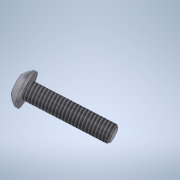
# Autodesk Inventor part: SCREW, BUTTON HD, P, 12.9, M4X0.7X18MM
Saved by Autodesk Inventor 2024.2 (Build 282272000, 272)
## iProperties
Manager: 100-31865
Category: _
Created: 2013-04-09
Material: Steel
Description: SCREW, BUTTON HD, P, 12.9, M4X0.7X18MM
Document SubType Name: Modeling
Designer: robr , Rob
Checked By: 2ATE9
Engr Approved By: R
User Status: Released
Density: 7.85 g/cm^3
Mfg Approved By: Rob.Roddy
Appearance: Plate
Part Number: SCREW, BUTTON HD, P, 12.9, M4X0.7X18MM
Mass: 2.32497 g
Surface Area: 3.53377 cm^2
Volume: 0.296174 cm^3
Control State: 0
Master: False
Checked Out: False
Shininess: 65.0
Length Units: 11269
Angle Units: 11279
Time Units: 11290
Mass Units: 11286
Length Display Precision: 4
Angle Display Precision: 2
Compacted: True
CN_SERVICEABLE: _
CN_MASS: 0.002378
CL_runCount: 1
FinishProperty: ToBeSet
FIRST_DESCRIPTION: SCREW, BUTTON HD, P, 12.9, M4X0.7X18MM
SECOND_DESCRIPTION: _
THIRD_DESCRIPTION: _
CN_DETAILER: -
CN_MFG_PART_NUM: FMPBHMA040070018
CN_MFG_NAME: -
STANDARDCLASSFLAG: R
CUSTOMERNUMBER: _
CN_DESIGNER: Rob.Roddy
PTC_WM_ITERATION: 3
PTC_WM_ORGANIZATION_ID: CLWC
PTC_WM_LIFECYCLE: CLWC_CAD_LC
Density: 7.86
Volumn: 1.0470389527034538
Area: 8.192112949038872
PropertySet Name: Model Information
Revision Number: 1
Subject: FMPBHMA040070018
Author: -
Keywords: -
Autodesk Inventor part; units mm, degrees
ref_plane "YZ Plane" through (0, 0, 0) normal (1, 0, 0) x (0, 1, 0)
ref_plane "XZ Plane" through (0, 0, 0) normal (0, 1, 0) x (-1, 0, 0)
ref_plane "XY Plane" through (0, 0, 0) normal (0, 0, 1) x (1, 0, 0)
sketch "Sketch1" plane through (0, 0, 0) normal (0, 0, 1) x (1, 0, 0)
  line L0 (0, -22.0606) -> (0, 6.3638) projected
  line L1 (0, 2.2) -> (2.25, 2.2)
  line L2 (3.8, 0) -> (3.8, 0.56)
  arc A0 (3.8, 0.56) -> (2.25, 2.2) centre (0, -1.479) ccw
  line L3 (3.8, 0) -> (2, 0)
  line L4 (2, 0) -> (2, -10)
  line L5 (2, -10) -> (0, -10)
  point P0 (0, 0)
  dimension "BoltDia" = 4
  dimension "HeadDia" = 7.6
  dimension "HeadHeight" = 2.2
  dimension "SideHeight" = 0.56
  dimension "TopFlatDia" = 4.5
  dimension "Length" = 10
  constraints: 10 end point, 5 perpendicular, 4 point on line, 2 point on circle, 1 centre point
  measures "BoltDia" diameter of L4 L0
  measures "HeadDia" diameter of L2 L0
  measures "HeadHeight" distance between parallel lines of L1 L3
  measures "SideHeight" distance of L2.start L2.end
  measures "TopFlatDia" diameter of L1.end L0
  measures "Length" distance of L3.end L4.end
revolve "Revolution1" add sketch "Sketch1" angle 360 about axis through (0, -10, 0) along (0, 1, 0)
sketch "Sketch2" plane through (0, 2.2, 0) normal (0, 1, 0) x (1, 0, 0)
  circle A0 centre (0, 0) radius 2.25 projected
  circle A1 centre (0, 0) radius 1.25 construction
  line L0 (-0.7217, 1.25) -> (0.7217, 1.25)
  line L1 (0.7217, 1.25) -> (1.4434, 0)
  line L2 (1.4434, 0) -> (0.7217, -1.25)
  line L3 (0.7217, -1.25) -> (-0.7217, -1.25)
  line L4 (-0.7217, -1.25) -> (-1.4434, 0)
  line L5 (-1.4434, 0) -> (-0.7217, 1.25)
  dimension "HexSize" = 2.5
  constraints: 12 end point, 6 tangent, 3 equal length, 2 parallel, 1 centre point, 1 coincident, 1 horizontal
  measures "HexSize" distance between parallel lines of L3 L0
extrude "Hex" cut sketch "Sketch2" against normal blind 1.3 contours L0 L1 L2 L3 L4 L5
thread "Thread1" size "M4x0.7" class "4g6g" standard "ANSI Metric M Profile" full length
chamfer "Chamfer1" distance 0.4 angle 45 1 edges at (-2, -10, 0)
equation "\"d11\" = 0.1 * BoltDia"
equation "\"d12\" = 0.1 * BoltDia"
equation "\"d17\" = HexSize"
body "Solid1"
